conecter to motor v1 (Autodesk Fusion 360 design; units mm, degrees)
Autodesk Fusion 360 part; units mm, degrees
sketch "Sketch1" plane through (0, 0, 0) normal (0, 0, 1) x (1, 0, 0)
  circle A0 centre (0, 0) radius 57.5
  circle A1 centre (0, 0) radius 65
  dimension "d1" = 115
  dimension "d2" = 130
  constraint coincident A0.centre A1.centre
  constraint concentric A0 A1
  measures "d1" diameter of A0
  measures "d2" diameter of A1
extrude "Extrude1" add sketch "Sketch1" along normal blind 20 contours A0 | A1
sketch "Sketch2" plane through (0, 0, 0) normal (0, 0, -1) x (-1, 0, 0)
  circle A0 centre (0, 0) radius 65
  circle A1 centre (0, 0) radius 57.5
  circle A2 centre (0, 0) radius 47.5
  dimension "d5" = 115
  dimension "d6" = 95
  constraint coincident A0.centre A1.centre
  constraint concentric A1 A2
  measures "d5" diameter of A1
  measures "d6" diameter of A2
extrude "Extrude2" cut sketch "Sketch2" against normal blind 3.2 contours A2
sketch "Sketch3" plane through (0, 0, 20) normal (0, 0, 1) x (1, 0, 0)
  circle A0 centre (0, 0) radius 65
  circle A1 centre (0, 0) radius 57.5
  line L0 (0, 0) -> (0, 57.5)
  dimension "d9" = 115
  constraint concentric A0 A1
  constraint coincident A0.centre A1.centre
  constraint vertical L0
  constraint coincident A1 L0.end
  measures "d9" diameter of A1
hole "Hole1" at (0, 57.5, 20) direction (0, 0, -1) diameter 8 end through all counterbore diameter 12 counterbore depth 9
pattern_circular "C-Pattern1" count 8 over 360 about axis through (0, 0, 1.75) along (0, 0, 1) of "Hole1"
sketch "Sketch4" plane through (0, 0, 20) normal (0, 0, 1) x (1, 0, 0)
  circle A0 centre (40.6586, 40.6586) radius 6
  circle A1 centre (57.5, 0) radius 6
  circle A2 centre (40.6586, -40.6586) radius 6
  circle A3 centre (0, -57.5) radius 6
  circle A4 centre (-40.6586, -40.6586) radius 6
  circle A5 centre (-57.5, 0) radius 6
  circle A6 centre (-40.6586, 40.6586) radius 6
  circle A7 centre (0, 57.5) radius 6
  circle A8 centre (0, 0) radius 65
  circle A9 centre (0, 0) radius 40
  dimension "d17" = 80
  constraint concentric A8 A9
  measures "d17" diameter of A9
extrude "Extrude3" cut sketch "Sketch4" against normal blind 17 contours A9
sketch "Sketch5" plane through (0, 0, 20) normal (0, 0, 1) x (1, 0, 0)
  circle A0 centre (0, 0) radius 40
  circle A1 centre (40.6586, 40.6586) radius 6
  circle A2 centre (57.5, 0) radius 6
  circle A3 centre (40.6586, -40.6586) radius 6
  circle A4 centre (0, -57.5) radius 6
  circle A5 centre (-40.6586, -40.6586) radius 6
  circle A6 centre (-57.5, 0) radius 6
  circle A7 centre (-40.6586, 40.6586) radius 6
  circle A8 centre (0, 57.5) radius 6
  circle A9 centre (0, 0) radius 65
  circle A10 centre (0, 0) radius 47.5
  dimension "d20" = 95
  constraint coincident A0.centre A9.centre
  measures "d20" diameter of A10
extrude "Extrude4" add sketch "Sketch5" along normal blind 80 contours A10
sketch "Sketch6" plane through (0, 0, 100) normal (0, 0, 1) x (1, 0, 0)
  circle A0 centre (0, 0) radius 40
  circle A1 centre (0, 0) radius 47.5
  circle A2 centre (0, 0) radius 65
  constraint concentric A0 A2
extrude "Extrude5" add sketch "Sketch6" along normal blind 20 contours A1 | A2
sketch "Sketch7" plane through (0, 0, 100) normal (0, 0, -1) x (-1, 0, 0)
  circle A0 centre (0, 0) radius 65
  circle A1 centre (0, 0) radius 47.5
  line L0 (0, 0) -> (0, 57.5)
  dimension "d25" = 57.5
  constraint coincident A0.centre A1.centre
  constraint vertical L0
  measures "d25" distance of A0.centre L0.end
hole "Hole2" at (0, 57.5, 100) direction (0, 0, 1) diameter 8 end through all counterbore diameter 12 counterbore depth 10
pattern_circular "C-Pattern2" count 8 over 360 about axis through (0, 0, 1.75) along (0, 0, 1) of "Hole2"
equation "d2 = 115 mm + 15 mm"
equation "d25 = ( 115 / 2 ) * 1 mm"
